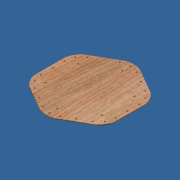
# Autodesk Inventor part: BottomBase_Full
Saved by Autodesk Inventor 2014 SP2 (Build 180246200, 246)
## iProperties
Created: 2015-02-19
Part Number: BottomBase_Full
Material: Holz (Birke)
Document SubType Name: Modeling
Designer: 4ndreas
Density: 0.55 g/cm^3
Appearance: Birke - natur - poliert
Author: 4ndreas
Autodesk Inventor part; units mm, degrees
ref_plane "YZ Plane" through (0, 0, 0) normal (1, 0, 0) x (0, 1, 0)
ref_plane "XZ Plane" through (0, 0, 0) normal (0, 1, 0) x (-1, 0, 0)
ref_plane "XY Plane" through (0, 0, 0) normal (0, 0, 1) x (1, 0, 0)
sketch "Skizze1" plane through (0, 0, 0) normal (0, 0, 1) x (1, 0, 0)
  circle A0 centre (60.6218, 105) radius 2.5
  circle A1 centre (-60.6218, 105) radius 2.5
  circle A2 centre (-121.2436, 0) radius 2.5
  circle A3 centre (-60.6218, -105) radius 2.5
  circle A4 centre (60.6218, -105) radius 2.5
  circle A5 centre (121.2436, 0) radius 2.5
  arc A6 (-66.5358, -13.0029) -> (-65.0733, -9.953) centre (-68.0388, -10.4066) ccw
  line L0 (-66.5358, -13.0029) -> (-66.8448, -13.1817)
  arc A7 (-66.8448, -13.1817) -> (-68.6633, -20.0004) centre (-40.9893, -23.7291) ccw
  line L1 (-68.6633, -20.0004) -> (-51.5367, -49.5845)
  arc A8 (-51.5367, -49.5845) -> (-44.7181, -51.4031) centre (-40.9893, -23.7291) ccw
  line L2 (-44.7181, -51.4031) -> (-44.4091, -51.2242)
  arc A9 (-41.036, -51.4747) -> (-44.4091, -51.2242) centre (-42.9061, -53.8205) ccw
  arc A10 (-41.036, -51.4747) -> (-65.0733, -9.953) centre (0, 0) ccw
  circle A11 centre (-63.1036, -36.5313) radius 3.3
  circle A12 centre (63.1888, -36.3837) radius 3.3
  circle A13 centre (-0.0852, 72.915) radius 3.3
  circle A14 centre (63.1036, 36.5313) radius 3.3
  circle A15 centre (0.0852, -72.915) radius 3.3
  circle A16 centre (-63.1888, 36.3837) radius 3.3
  arc A17 (131.2436, 25.0172) -> (128.4541, 26.8548) centre (129.2436, 25.0172) ccw
  line L3 (131.2436, 25.0172) -> (131.2436, -25.0172)
  arc A18 (128.4541, -26.8548) -> (131.2436, -25.0172) centre (129.2436, -25.0172) ccw
  arc A19 (128.4541, -26.8548) -> (126.2436, -26.4) centre (126.2436, -32) ccw
  line L4 (126.2436, -26.4) -> (110.2436, -26.4) construction
  arc A20 (110.2436, -26.4) -> (104.6436, -32) centre (110.2436, -32) ccw construction
  line L5 (104.6436, -32) -> (104.6436, -40.5551) construction
  arc A21 (98.0436, -44.3656) -> (104.6436, -40.5551) centre (100.2436, -40.5551) ccw construction
  line L6 (98.0436, -44.3656) -> (92.5532, -41.1958) construction
  arc A22 (92.5532, -41.1958) -> (84.9034, -43.2455) centre (89.7532, -46.0455) ccw construction
  line L7 (84.9034, -43.2455) -> (79.9034, -51.9058) construction
  arc A23 (79.9034, -51.9058) -> (81.9532, -59.5555) centre (84.7532, -54.7058) ccw construction
  line L8 (81.9532, -59.5555) -> (87.4436, -62.7254) construction
  arc A24 (87.4436, -70.3464) -> (87.4436, -62.7254) centre (85.2436, -66.5359) ccw construction
  line L9 (87.4436, -70.3464) -> (80.0346, -74.624) construction
  arc A25 (80.0346, -74.624) -> (77.9848, -82.2737) centre (82.8346, -79.4737) ccw construction
  line L10 (77.9848, -82.2737) -> (85.9848, -96.1301) construction
  arc A26 (85.9848, -96.1301) -> (87.4839, -97.8171) centre (90.8346, -93.3301) ccw
  arc A27 (87.2873, -101.1517) -> (87.4839, -97.8171) centre (86.2873, -99.4196) ccw
  line L11 (87.2873, -101.1517) -> (43.9563, -126.1688)
  arc A28 (40.9701, -124.6719) -> (43.9563, -126.1688) centre (42.9563, -124.4368) ccw
  arc A29 (40.9701, -124.6719) -> (40.2587, -122.5301) centre (35.409, -125.3301) ccw
  line L12 (40.2587, -122.5301) -> (32.2587, -108.6737) construction
  arc A30 (32.2587, -108.6737) -> (24.609, -106.624) centre (27.409, -111.4737) ccw construction
  line L13 (24.609, -106.624) -> (17.2, -110.9015) construction
  arc A31 (10.6, -107.091) -> (17.2, -110.9015) centre (15, -107.091) ccw construction
  line L14 (10.6, -107.091) -> (10.6, -100.7513) construction
  arc A32 (10.6, -100.7513) -> (5, -95.1513) centre (5, -100.7513) ccw construction
  line L15 (5, -95.1513) -> (-5, -95.1513) construction
  arc A33 (-5, -95.1513) -> (-10.6, -100.7513) centre (-5, -100.7513) ccw construction
  line L16 (-10.6, -100.7513) -> (-10.6, -107.091) construction
  arc A34 (-17.2, -110.9015) -> (-10.6, -107.091) centre (-15, -107.091) ccw construction
  line L17 (-17.2, -110.9015) -> (-24.609, -106.624) construction
  arc A35 (-24.609, -106.624) -> (-32.2587, -108.6737) centre (-27.409, -111.4737) ccw construction
  line L18 (-32.2587, -108.6737) -> (-40.2587, -122.5301) construction
  arc A36 (-40.2587, -122.5301) -> (-40.9701, -124.6719) centre (-35.409, -125.3301) ccw
  arc A37 (-43.9563, -126.1688) -> (-40.9701, -124.6719) centre (-42.9563, -124.4368) ccw
  line L19 (-43.9563, -126.1688) -> (-87.2873, -101.1517)
  arc A38 (-87.4839, -97.8171) -> (-87.2873, -101.1517) centre (-86.2873, -99.4196) ccw
  arc A39 (-87.4839, -97.8171) -> (-85.9848, -96.1301) centre (-90.8346, -93.3301) ccw
  line L20 (-85.9848, -96.1301) -> (-77.9848, -82.2737) construction
  arc A40 (-77.9848, -82.2737) -> (-80.0346, -74.624) centre (-82.8346, -79.4737) ccw construction
  line L21 (-80.0346, -74.624) -> (-87.4436, -70.3464) construction
  arc A41 (-87.4436, -62.7254) -> (-87.4436, -70.3464) centre (-85.2436, -66.5359) ccw construction
  line L22 (-87.4436, -62.7254) -> (-81.9532, -59.5555) construction
  arc A42 (-81.9532, -59.5555) -> (-79.9034, -51.9058) centre (-84.7532, -54.7058) ccw construction
  line L23 (-79.9034, -51.9058) -> (-84.9034, -43.2455) construction
  arc A43 (-84.9034, -43.2455) -> (-92.5532, -41.1958) centre (-89.7532, -46.0455) ccw construction
  line L24 (-92.5532, -41.1958) -> (-98.0436, -44.3656) construction
  arc A44 (-104.6436, -40.5551) -> (-98.0436, -44.3656) centre (-100.2436, -40.5551) ccw construction
  line L25 (-104.6436, -40.5551) -> (-104.6436, -32) construction
  arc A45 (-104.6436, -32) -> (-110.2436, -26.4) centre (-110.2436, -32) ccw construction
  line L26 (-110.2436, -26.4) -> (-126.2436, -26.4) construction
  arc A46 (-126.2436, -26.4) -> (-128.4541, -26.8548) centre (-126.2436, -32) ccw
  arc A47 (-131.2436, -25.0172) -> (-128.4541, -26.8548) centre (-129.2436, -25.0172) ccw
  line L27 (-131.2436, -25.0172) -> (-131.2436, 25.0172)
  arc A48 (-128.4541, 26.8548) -> (-131.2436, 25.0172) centre (-129.2436, 25.0172) ccw
  arc A49 (-128.4541, 26.8548) -> (-126.2436, 26.4) centre (-126.2436, 32) ccw
  line L28 (-126.2436, 26.4) -> (-110.2436, 26.4) construction
  arc A50 (-110.2436, 26.4) -> (-104.6436, 32) centre (-110.2436, 32) ccw construction
  line L29 (-104.6436, 32) -> (-104.6436, 40.5551) construction
  arc A51 (-98.0436, 44.3656) -> (-104.6436, 40.5551) centre (-100.2436, 40.5551) ccw construction
  line L30 (-98.0436, 44.3656) -> (-92.5532, 41.1958) construction
  arc A52 (-92.5532, 41.1958) -> (-84.9034, 43.2455) centre (-89.7532, 46.0455) ccw construction
  line L31 (-84.9034, 43.2455) -> (-79.9034, 51.9058) construction
  arc A53 (-79.9034, 51.9058) -> (-81.9532, 59.5555) centre (-84.7532, 54.7058) ccw construction
  line L32 (-81.9532, 59.5555) -> (-87.4436, 62.7254) construction
  arc A54 (-87.4436, 70.3464) -> (-87.4436, 62.7254) centre (-85.2436, 66.5359) ccw construction
  line L33 (-87.4436, 70.3464) -> (-80.0346, 74.624) construction
  arc A55 (-80.0346, 74.624) -> (-77.9848, 82.2737) centre (-82.8346, 79.4737) ccw construction
  line L34 (-77.9848, 82.2737) -> (-85.9848, 96.1301) construction
  arc A56 (-85.9848, 96.1301) -> (-87.4839, 97.8171) centre (-90.8346, 93.3301) ccw
  arc A57 (-87.2873, 101.1517) -> (-87.4839, 97.8171) centre (-86.2873, 99.4196) ccw
  line L35 (-87.2873, 101.1517) -> (-43.9563, 126.1688)
  arc A58 (-40.9701, 124.6719) -> (-43.9563, 126.1688) centre (-42.9563, 124.4368) ccw
  arc A59 (-40.9701, 124.6719) -> (-40.2587, 122.5301) centre (-35.409, 125.3301) ccw
  line L36 (-40.2587, 122.5301) -> (-32.2587, 108.6737)
  arc A60 (-32.2587, 108.6737) -> (-24.609, 106.624) centre (-27.409, 111.4737) ccw
  line L37 (-24.609, 106.624) -> (-17.2, 110.9015) construction
  arc A61 (-10.6, 107.091) -> (-17.2, 110.9015) centre (-15, 107.091) ccw construction
  line L38 (-10.6, 107.091) -> (-10.6, 100.7513)
  arc A62 (-10.6, 100.7513) -> (-5, 95.1513) centre (-5, 100.7513) ccw construction
  line L39 (-5, 95.1513) -> (5, 95.1513) construction
  arc A63 (5, 95.1513) -> (10.6, 100.7513) centre (5, 100.7513) ccw construction
  line L40 (10.6, 100.7513) -> (10.6, 107.091)
  arc A64 (17.2, 110.9015) -> (10.6, 107.091) centre (15, 107.091) ccw construction
  line L41 (17.2, 110.9015) -> (24.609, 106.624) construction
  arc A65 (24.609, 106.624) -> (32.2587, 108.6737) centre (27.409, 111.4737) ccw construction
  line L42 (32.2587, 108.6737) -> (40.2587, 122.5301) construction
  arc A66 (40.2587, 122.5301) -> (40.9701, 124.6719) centre (35.409, 125.3301) ccw
  arc A67 (43.9563, 126.1688) -> (40.9701, 124.6719) centre (42.9563, 124.4368) ccw
  line L43 (43.9563, 126.1688) -> (87.2873, 101.1517)
  arc A68 (87.4839, 97.8171) -> (87.2873, 101.1517) centre (86.2873, 99.4196) ccw
  arc A69 (87.4839, 97.8171) -> (85.9848, 96.1301) centre (90.8346, 93.3301) ccw
  line L44 (85.9848, 96.1301) -> (77.9848, 82.2737) construction
  arc A70 (77.9848, 82.2737) -> (80.0346, 74.624) centre (82.8346, 79.4737) ccw construction
  line L45 (80.0346, 74.624) -> (87.4436, 70.3464) construction
  arc A71 (87.4436, 62.7254) -> (87.4436, 70.3464) centre (85.2436, 66.5359) ccw construction
  line L46 (87.4436, 62.7254) -> (81.9532, 59.5555) construction
  arc A72 (81.9532, 59.5555) -> (79.9034, 51.9058) centre (84.7532, 54.7058) ccw construction
  line L47 (79.9034, 51.9058) -> (84.9034, 43.2455) construction
  arc A73 (84.9034, 43.2455) -> (92.5532, 41.1958) centre (89.7532, 46.0455) ccw construction
  line L48 (92.5532, 41.1958) -> (98.0436, 44.3656) construction
  arc A74 (104.6436, 40.5551) -> (98.0436, 44.3656) centre (100.2436, 40.5551) ccw construction
  line L49 (104.6436, 40.5551) -> (104.6436, 32) construction
  arc A75 (104.6436, 32) -> (110.2436, 26.4) centre (110.2436, 32) ccw construction
  line L50 (110.2436, 26.4) -> (126.2436, 26.4) construction
  arc A76 (126.2436, 26.4) -> (128.4541, 26.8548) centre (126.2436, 32) ccw
  arc A77 (80.3346, -75.1436) -> (78.5045, -81.9737) centre (82.8346, -79.4737) ccw construction
  line L51 (80.3346, -75.1436) -> (87.7436, -70.866) construction
  arc A78 (87.7436, -70.866) -> (87.7436, -62.2058) centre (85.2436, -66.5359) ccw construction
  line L52 (87.7436, -62.2058) -> (82.2532, -59.0359) construction
  arc A79 (80.423, -52.2058) -> (82.2532, -59.0359) centre (84.7532, -54.7058) ccw construction
  line L53 (80.423, -52.2058) -> (85.423, -43.5455) construction
  arc A80 (92.2532, -41.7154) -> (85.423, -43.5455) centre (89.7532, -46.0455) ccw construction
  line L54 (92.2532, -41.7154) -> (97.7436, -44.8853) construction
  arc A81 (97.7436, -44.8853) -> (105.2436, -40.5551) centre (100.2436, -40.5551) ccw construction
  line L55 (105.2436, -40.5551) -> (105.2436, -32) construction
  arc A82 (110.2436, -27) -> (105.2436, -32) centre (110.2436, -32) ccw construction
  line L56 (110.2436, -27) -> (126.2436, -27) construction
  arc A83 (131.2436, -32) -> (126.2436, -27) centre (126.2436, -32) ccw
  line L57 (131.2436, -32) -> (131.2436, -50)
  line L58 (131.2436, -50) -> (127.9756, -62.3397)
  line L59 (127.9756, -62.3397) -> (117.9756, -79.6603)
  line L60 (117.9756, -79.6603) -> (108.923, -88.6603)
  line L61 (108.923, -88.6603) -> (93.3346, -97.6603)
  arc A84 (86.5045, -95.8301) -> (93.3346, -97.6603) centre (90.8346, -93.3301) ccw
  line L62 (86.5045, -95.8301) -> (78.5045, -81.9737) construction
  circle A85 centre (114.3154, -66) radius 5.5 construction
  circle A86 centre (91.5833, -52.8756) radius 5.5 construction
  circle A87 centre (93.9638, -85.75) radius 5.5 construction
  circle A88 centre (121.2436, -38.5) radius 5.5 construction
  arc A89 (105.2436, 32) -> (110.2436, 27) centre (110.2436, 32) ccw construction
  line L63 (105.2436, 32) -> (105.2436, 40.5551) construction
  arc A90 (105.2436, 40.5551) -> (97.7436, 44.8853) centre (100.2436, 40.5551) ccw construction
  line L64 (97.7436, 44.8853) -> (92.2532, 41.7154) construction
  arc A91 (85.423, 43.5455) -> (92.2532, 41.7154) centre (89.7532, 46.0455) ccw construction
  line L65 (85.423, 43.5455) -> (80.423, 52.2058) construction
  arc A92 (82.2532, 59.0359) -> (80.423, 52.2058) centre (84.7532, 54.7058) ccw construction
  line L66 (82.2532, 59.0359) -> (87.7436, 62.2058) construction
  arc A93 (87.7436, 62.2058) -> (87.7436, 70.866) centre (85.2436, 66.5359) ccw construction
  line L67 (87.7436, 70.866) -> (80.3346, 75.1436) construction
  arc A94 (78.5045, 81.9737) -> (80.3346, 75.1436) centre (82.8346, 79.4737) ccw construction
  line L68 (78.5045, 81.9737) -> (86.5045, 95.8301) construction
  arc A95 (93.3346, 97.6603) -> (86.5045, 95.8301) centre (90.8346, 93.3301) ccw
  line L69 (93.3346, 97.6603) -> (108.923, 88.6603)
  line L70 (108.923, 88.6603) -> (117.9756, 79.6603)
  line L71 (117.9756, 79.6603) -> (127.9756, 62.3397)
  line L72 (127.9756, 62.3397) -> (131.2436, 50)
  line L73 (131.2436, 50) -> (131.2436, 32)
  arc A96 (126.2436, 27) -> (131.2436, 32) centre (126.2436, 32) ccw
  line L74 (126.2436, 27) -> (110.2436, 27) construction
  circle A97 centre (114.3154, 66) radius 5.5 construction
  circle A98 centre (91.5833, 52.8756) radius 5.5 construction
  circle A99 centre (121.2436, 38.5) radius 5.5 construction
  circle A100 centre (93.9638, 85.75) radius 5.5 construction
  arc A101 (24.909, 107.1436) -> (31.7391, 108.9737) centre (27.409, 111.4737) ccw construction
  line L75 (24.909, 107.1436) -> (17.5, 111.4212) construction
  arc A102 (17.5, 111.4212) -> (10, 107.091) centre (15, 107.091) ccw construction
  line L76 (10, 107.091) -> (10, 100.7513)
  arc A103 (5, 95.7513) -> (10, 100.7513) centre (5, 100.7513) ccw construction
  line L77 (5, 95.7513) -> (-5, 95.7513) construction
  arc A104 (-10, 100.7513) -> (-5, 95.7513) centre (-5, 100.7513) ccw construction
  line L78 (-10, 100.7513) -> (-10, 107.091)
  arc A105 (-10, 107.091) -> (-17.5, 111.4212) centre (-15, 107.091) ccw construction
  line L79 (-17.5, 111.4212) -> (-24.909, 107.1436) construction
  arc A106 (-31.7391, 108.9737) -> (-24.909, 107.1436) centre (-27.409, 111.4737) ccw
  line L80 (-31.7391, 108.9737) -> (-39.7391, 122.8301)
  arc A107 (-37.909, 129.6603) -> (-39.7391, 122.8301) centre (-35.409, 125.3301) ccw
  line L81 (-37.909, 129.6603) -> (-22.3205, 138.6603)
  line L82 (-22.3205, 138.6603) -> (-10, 142)
  line L83 (-10, 142) -> (10, 142)
  line L84 (10, 142) -> (22.3205, 138.6603)
  line L85 (22.3205, 138.6603) -> (37.909, 129.6603)
  arc A108 (39.7391, 122.8301) -> (37.909, 129.6603) centre (35.409, 125.3301) ccw
  line L86 (39.7391, 122.8301) -> (31.7391, 108.9737) construction
  circle A109 centre (0, 132) radius 5.5 construction
  circle A110 centre (0, 105.7513) radius 5.5 construction
  circle A111 centre (27.2798, 124.25) radius 5.5 construction
  circle A112 centre (-27.2798, 124.25) radius 5.5 construction
  arc A113 (-80.3346, 75.1436) -> (-78.5045, 81.9737) centre (-82.8346, 79.4737) ccw construction
  line L87 (-80.3346, 75.1436) -> (-87.7436, 70.866) construction
  arc A114 (-87.7436, 70.866) -> (-87.7436, 62.2058) centre (-85.2436, 66.5359) ccw construction
  line L88 (-87.7436, 62.2058) -> (-82.2532, 59.0359) construction
  arc A115 (-80.423, 52.2058) -> (-82.2532, 59.0359) centre (-84.7532, 54.7058) ccw construction
  line L89 (-80.423, 52.2058) -> (-85.423, 43.5455) construction
  arc A116 (-92.2532, 41.7154) -> (-85.423, 43.5455) centre (-89.7532, 46.0455) ccw construction
  line L90 (-92.2532, 41.7154) -> (-97.7436, 44.8853) construction
  arc A117 (-97.7436, 44.8853) -> (-105.2436, 40.5551) centre (-100.2436, 40.5551) ccw construction
  line L91 (-105.2436, 40.5551) -> (-105.2436, 32) construction
  arc A118 (-110.2436, 27) -> (-105.2436, 32) centre (-110.2436, 32) ccw construction
  line L92 (-110.2436, 27) -> (-126.2436, 27) construction
  arc A119 (-131.2436, 32) -> (-126.2436, 27) centre (-126.2436, 32) ccw
  line L93 (-131.2436, 32) -> (-131.2436, 50)
  line L94 (-131.2436, 50) -> (-127.9756, 62.3397)
  line L95 (-127.9756, 62.3397) -> (-117.9756, 79.6603)
  line L96 (-117.9756, 79.6603) -> (-108.923, 88.6603)
  line L97 (-108.923, 88.6603) -> (-93.3346, 97.6603)
  arc A120 (-86.5045, 95.8301) -> (-93.3346, 97.6603) centre (-90.8346, 93.3301) ccw
  line L98 (-86.5045, 95.8301) -> (-78.5045, 81.9737) construction
  circle A121 centre (-114.3154, 66) radius 5.5 construction
  circle A122 centre (-91.5833, 52.8756) radius 5.5 construction
  circle A123 centre (-93.9638, 85.75) radius 5.5 construction
  circle A124 centre (-121.2436, 38.5) radius 5.5 construction
  arc A125 (-105.2436, -32) -> (-110.2436, -27) centre (-110.2436, -32) ccw construction
  line L99 (-105.2436, -32) -> (-105.2436, -40.5551) construction
  arc A126 (-105.2436, -40.5551) -> (-97.7436, -44.8853) centre (-100.2436, -40.5551) ccw construction
  line L100 (-97.7436, -44.8853) -> (-92.2532, -41.7154) construction
  arc A127 (-85.423, -43.5455) -> (-92.2532, -41.7154) centre (-89.7532, -46.0455) ccw construction
  line L101 (-85.423, -43.5455) -> (-80.423, -52.2058) construction
  arc A128 (-82.2532, -59.0359) -> (-80.423, -52.2058) centre (-84.7532, -54.7058) ccw construction
  line L102 (-82.2532, -59.0359) -> (-87.7436, -62.2058) construction
  arc A129 (-87.7436, -62.2058) -> (-87.7436, -70.866) centre (-85.2436, -66.5359) ccw construction
  line L103 (-87.7436, -70.866) -> (-80.3346, -75.1436) construction
  arc A130 (-78.5045, -81.9737) -> (-80.3346, -75.1436) centre (-82.8346, -79.4737) ccw construction
  line L104 (-78.5045, -81.9737) -> (-86.5045, -95.8301) construction
  arc A131 (-93.3346, -97.6603) -> (-86.5045, -95.8301) centre (-90.8346, -93.3301) ccw
  line L105 (-93.3346, -97.6603) -> (-108.923, -88.6603)
  line L106 (-108.923, -88.6603) -> (-117.9756, -79.6603)
  line L107 (-117.9756, -79.6603) -> (-127.9756, -62.3397)
  line L108 (-127.9756, -62.3397) -> (-131.2436, -50)
  line L109 (-131.2436, -50) -> (-131.2436, -32)
  arc A132 (-126.2436, -27) -> (-131.2436, -32) centre (-126.2436, -32) ccw
  line L110 (-126.2436, -27) -> (-110.2436, -27) construction
  circle A133 centre (-114.3154, -66) radius 5.5 construction
  circle A134 centre (-91.5833, -52.8756) radius 5.5 construction
  circle A135 centre (-121.2436, -38.5) radius 5.5 construction
  circle A136 centre (-93.9638, -85.75) radius 5.5 construction
  arc A137 (-24.909, -107.1436) -> (-31.7391, -108.9737) centre (-27.409, -111.4737) ccw construction
  line L111 (-24.909, -107.1436) -> (-17.5, -111.4212) construction
  arc A138 (-17.5, -111.4212) -> (-10, -107.091) centre (-15, -107.091) ccw construction
  line L112 (-10, -107.091) -> (-10, -100.7513) construction
  arc A139 (-5, -95.7513) -> (-10, -100.7513) centre (-5, -100.7513) ccw construction
  line L113 (-5, -95.7513) -> (5, -95.7513) construction
  arc A140 (10, -100.7513) -> (5, -95.7513) centre (5, -100.7513) ccw construction
  line L114 (10, -100.7513) -> (10, -107.091) construction
  arc A141 (10, -107.091) -> (17.5, -111.4212) centre (15, -107.091) ccw construction
  line L115 (17.5, -111.4212) -> (24.909, -107.1436) construction
  arc A142 (31.7391, -108.9737) -> (24.909, -107.1436) centre (27.409, -111.4737) ccw construction
  line L116 (31.7391, -108.9737) -> (39.7391, -122.8301) construction
  arc A143 (37.909, -129.6603) -> (39.7391, -122.8301) centre (35.409, -125.3301) ccw
  line L117 (37.909, -129.6603) -> (22.3205, -138.6603)
  line L118 (22.3205, -138.6603) -> (10, -142)
  line L119 (10, -142) -> (-10, -142)
  line L120 (-10, -142) -> (-22.3205, -138.6603)
  line L121 (-22.3205, -138.6603) -> (-37.909, -129.6603)
  arc A144 (-39.7391, -122.8301) -> (-37.909, -129.6603) centre (-35.409, -125.3301) ccw
  line L122 (-39.7391, -122.8301) -> (-31.7391, -108.9737) construction
  circle A145 centre (0, -132) radius 5.5 construction
  circle A146 centre (0, -105.7513) radius 5.5 construction
  circle A147 centre (-27.2798, -124.25) radius 5.5 construction
  circle A148 centre (27.2798, -124.25) radius 5.5 construction
  line L123 (-131.2436, -25.0172) -> (-131.2436, -32)
  line L124 (-93.3346, -97.6603) -> (-87.2873, -101.1517)
  line L125 (-43.9563, -126.1688) -> (-37.909, -129.6603)
  line L126 (37.909, -129.6603) -> (43.9563, -126.1688)
  line L127 (87.2873, -101.1517) -> (93.3346, -97.6603)
  line L128 (131.2436, -32) -> (131.2436, -25.0172)
  line L129 (131.2436, 25.0172) -> (131.2436, 32)
  line L130 (93.3346, 97.6603) -> (87.2873, 101.1517)
  line L131 (43.9563, 126.1688) -> (37.909, 129.6603)
  line L132 (-37.909, 129.6603) -> (-43.9563, 126.1688)
  line L133 (-87.2873, 101.1517) -> (-93.3346, 97.6603)
  line L134 (-131.2436, 32) -> (-131.2436, 25.0172)
  circle A149 centre (-27.2798, 124.25) radius 2.5
  circle A150 centre (0, 105.7513) radius 2.5
  circle A151 centre (0, 132) radius 2.5
  circle A152 centre (27.2798, 124.25) radius 2.5
  circle A153 centre (-121.2436, 38.5) radius 2.5
  circle A154 centre (-91.5833, 52.8756) radius 2.5
  circle A155 centre (-114.3154, 66) radius 2.5
  circle A156 centre (-93.9638, 85.75) radius 2.5
  circle A157 centre (-93.9638, -85.75) radius 2.5
  circle A158 centre (-91.5833, -52.8756) radius 2.5
  circle A159 centre (-114.3154, -66) radius 2.5
  circle A160 centre (-121.2436, -38.5) radius 2.5
  circle A161 centre (27.2798, -124.25) radius 2.5
  circle A162 centre (0, -105.7513) radius 2.5
  circle A163 centre (0, -132) radius 2.5
  circle A164 centre (-27.2798, -124.25) radius 2.5
  circle A165 centre (121.2436, -38.5) radius 2.5
  circle A166 centre (91.5833, -52.8756) radius 2.5
  circle A167 centre (114.3154, -66) radius 2.5
  circle A168 centre (93.9638, -85.75) radius 2.5
  circle A169 centre (93.9638, 85.75) radius 2.5
  circle A170 centre (91.5833, 52.8756) radius 2.5
  circle A171 centre (114.3154, 66) radius 2.5
  circle A172 centre (121.2436, 38.5) radius 2.5
  point P0 (0, 0)
  dimension "d3" = 360
  constraints: 270 end point, 230 point on circle, 173 centre point, 22 vertical, 14 horizontal, 14 tangent, 8 collinear, 4 equal radius, 670 other
extrude "Extrusion1" add sketch "Skizze1" along normal blind 3 contours A1 | L3 L128 L57 L58 L59 L60 L61 L127 L11 L126 L117 L118 L119 L120 L121 L125 L19 L124 L105 L106 L107 L108 L109 L123 L27 L134 L93 L94 L95 L96 L97 L133 L35 L132 L81 L82 L83 L84 L85 L131 L43 L130 L69 L70 L71 L72 L73 L129
sketch "Skizze2" plane through (0, 0, 3) normal (0, 0, 1) x (1, 0, 0)
  arc A0 (-41.036, -51.4747) -> (-65.0733, -9.953) centre (0, 0) ccw projected
  arc A1 (-41.036, -51.4747) -> (-44.4091, -51.2242) centre (-42.9061, -53.8205) ccw projected
  line L0 (-44.4091, -51.2242) -> (-44.7181, -51.4031) projected
  arc A2 (-51.5367, -49.5845) -> (-44.7181, -51.4031) centre (-40.9893, -23.7291) ccw projected
  line L1 (-51.5367, -49.5845) -> (-68.6633, -20.0004) projected
  arc A3 (-66.8448, -13.1817) -> (-68.6633, -20.0004) centre (-40.9893, -23.7291) ccw projected
  line L2 (-66.8448, -13.1817) -> (-66.5358, -13.0029) projected
  arc A4 (-66.5358, -13.0029) -> (-65.0733, -9.953) centre (-68.0388, -10.4066) ccw projected
  circle A5 centre (-63.1888, 36.3837) radius 3.3 projected
  circle A6 centre (0.0852, -72.915) radius 3.3 projected
  circle A7 centre (63.1036, 36.5313) radius 3.3 projected
  circle A8 centre (-0.0852, 72.915) radius 3.3 projected
  circle A9 centre (63.1888, -36.3837) radius 3.3 projected
  circle A10 centre (-63.1036, -36.5313) radius 3.3 projected
extrude "Extrusion2" add sketch "Skizze2" against normal up to surface (3 mm away)
